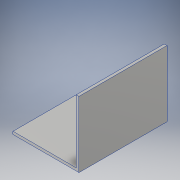
# Autodesk Inventor part: ARM_068_NewLongShaftMountFlipped
Saved by Autodesk Inventor 2018 (Build 220112000, 112)
## iProperties
Created: 2020-02-11
Part Number: ARM_068_NewLongShaftMountFlipped
Material: Aluminum 6061
Document SubType Name: Modeling
Designer: user
Mass: 129.97 g
Surface Area: 319.153 cm^2
Volume: 48.137 cm^3
Density: 2.7 g/cm^3
Appearance: Aluminum - Flat
Author: user
Autodesk Inventor part; units mm, degrees
ref_plane "YZ Plane" through (0, 0, 0) normal (1, 0, 0) x (0, 1, 0)
ref_plane "XZ Plane" through (0, 0, 0) normal (0, 1, 0) x (-1, 0, 0)
ref_plane "XY Plane" through (0, 0, 0) normal (0, 0, 1) x (1, 0, 0)
sketch "Sketch1" plane through (0, 0, 0) normal (0, 0, 1) x (1, 0, 0)
  line L0 (0, 0) -> (76.2, 0)
  line L1 (76.2, 0) -> (76.2, 76.2)
  line L2 (76.2, 76.2) -> (0, 76.2)
  line L3 (0, 3.175) -> (0, 0)
  line L4 (3.175, 3.175) -> (73.025, 3.175)
  line L5 (73.025, 3.175) -> (73.025, 73.025)
  line L6 (3.175, 3.175) -> (0, 3.175)
  line L7 (73.025, 73.025) -> (73.025, 76.2)
  dimension "d0" = 76.2
  dimension "d1" = 76.2
  constraints: 16 end point, 2 horizontal, 2 parallel, 2 perpendicular, 1 point on line, 1 vertical, 1 other
  measures "d0" distance of L2.end L1.end
  measures "d1" distance of L1.end L0.end
extrude "Extrusion1" add sketch "Sketch1" along normal blind 101.6
sketch "Sketch2" plane through (0, 0, 0) normal (0, -1, 0) x (1, 0, 0)
  line L0 (0, 101.6) -> (76.2, 101.6) projected
  line L1 (0, 0) -> (0, 101.6) projected
  point P0 (20.6375, 20.6375)
  dimension "d5" = 80.9625
  dimension "d6" = 20.6375
  dimension "d14" = 101.6
  measures "d5" distance from line of L0 point (20.637, 20.637)
  measures "d6" distance from line of L1 point (20.637, 20.637)
  measures "d14" distance of L1.start L0.start
hole "Hole1" at (20.6375, 0, 20.6375) direction (0, 1, 0) diameter 28.575 depth 25.4 tip angle 118
body "Solid1"
